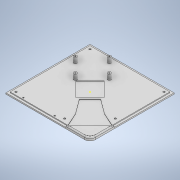
# Autodesk Inventor part: Box_Walls_2
Saved by Autodesk Inventor 2022 (Build 260153000, 153)
## iProperties
Created: 2023-02-27
Part Number: Box_Walls_2
Material: Generic
Document SubType Name: Modeling
Designer: zarek
Density: 1 g/cm^3
Appearance: Default
Author: zarek
Autodesk Inventor part; units mm, degrees
ref_plane "YZ Plane" through (0, 0, 0) normal (1, 0, 0) x (0, 1, 0)
ref_plane "XZ Plane" through (0, 0, 0) normal (0, 1, 0) x (-1, 0, 0)
sketch "Sketch1" plane through (0, 0, 0) normal (0, 1, 0) x (-1, 0, 0)
  line L0 (101.6, -101.6) -> (-101.6, -101.6)
  line L1 (-101.6, -101.6) -> (-101.6, 101.6)
  line L2 (-101.6, 101.6) -> (101.6, 101.6)
  line L3 (101.6, 101.6) -> (101.6, -101.6)
  line L4 (96.6, -96.6) -> (-96.6, -96.6)
  line L5 (-96.6, -96.6) -> (-96.6, 96.6)
  line L6 (-96.6, 96.6) -> (96.6, 96.6)
  line L7 (96.6, 96.6) -> (96.6, -96.6)
  line L8 (101.6, 101.6) -> (-40.4, 101.6)
  circle A0 centre (0, 0) radius 88.9
  circle A1 centre (0, 0) radius 109.3376
  line L9 (-40.4, 101.6) -> (-101.6, 40.4)
  line L10 (-45.4, 101.6) -> (-101.6, 45.4)
  line L11 (96.6, 96.6) -> (96.6, 101.6)
  line L12 (-45.4, 101.6) -> (-35.4, 101.6)
  line L13 (-35.4, 101.6) -> (-35.4, 96.6)
  line L14 (-35.4, 96.6) -> (-45.4, 96.6)
  line L15 (-45.4, 96.6) -> (-45.4, 101.6)
  line L16 (-45.4, 101.6) -> (-43.114, 101.6)
  line L17 (-43.114, 101.6) -> (-43.114, 96.6)
  line L18 (-43.114, 96.6) -> (-45.4, 96.6)
  line L19 (-45.4, 96.6) -> (-45.4, 101.6)
  line L20 (-96.6, 45.4) -> (-101.6, 45.4)
  line L21 (-101.6, 45.4) -> (-101.6, 43.114)
  line L22 (-101.6, 43.114) -> (-96.6, 43.114)
  line L23 (-96.6, 43.114) -> (-96.6, 45.4)
  point P0 (96.6, 51.2168)
  point P1 (101.6, 40.4)
  point P2 (101.6, -40.4)
  point P3 (96.6, -51.2168)
  point P4 (-96.6, 45.4)
  point P5 (-45.4, 96.6)
  dimension "d0" = 203.2
  dimension "d1" = 203.2
  dimension "d2" = 101.6
  dimension "d3" = 101.6
  dimension "d4" = 5
  dimension "d5" = 5
  dimension "d6" = 5
  dimension "d7" = 5
  dimension "d10" = 142
  dimension "d12" = 61.2
  dimension "d14" = 177.8
  dimension "d15" = 5
  dimension "d16" = 5
  dimension "d17" = 10
  dimension "d86" = 2.286
  dimension "d87" = 2.286
  constraints: 48 end point, 11 parallel, 10 point on line, 6 perpendicular, 5 horizontal, 2 centre point, 2 coincident, 2 point on circle
  measures "d0" distance between parallel lines of L2 L0
  measures "d1" distance between parallel lines of L1 L3
  measures "d2" distance from line of L0 point (0, 0)
  measures "d3" distance from line of L1 point (0, 0)
  measures "d4" distance between parallel lines of L4 L0
  measures "d5" distance between parallel lines of L1 L5
  measures "d6" distance between parallel lines of L2 L6
  measures "d7" distance between parallel lines of L3 L7
  measures "d10" distance of L2.end L8.end
  measures "d12" distance from line of L1 L8.end
  measures "d14" diameter of A0
  measures "d15" distance of L10.end L9.end
  measures "d16" distance of L10.start L8.end
  measures "d17" distance of L13.end L14.end
  measures "d86" distance of L17.end L18.end
  measures "d87" distance of L21.end L20.end
extrude "Extrusion1" add sketch "Sketch1" along normal blind 5 contours L0 A1 L4 L7 L3 | L0 A1 L4 | A1 L7 L3 | L0 L1 A1 L5 L4 | A1 L7 L4 | L4 A1 L5 L9 L6 L7 | A1 L7 L11 L2 L3 | L4 L5 A1 | A1 L6 L7 | L1 L9 L22 L5 A1 | L11 L6 A1 L2 | L6 L13 L2 A1 | L1 L22 A1 | A1 L22 L9 | L22 L9 L5 | L6 L17 L9 L2 L13 | L1 L20 A1 L22 | A1 L20 L9 L22 | L20 A1 L10 L5 | L5 L10 L6 L9 | A1 L17 L2 | L9 L17 A1 | L6 L9 L17 | L1 L2 L10 A1 L6 L5 | L10 A1 L20 | L10 A1 L5 | L5 A1 L6 L10 | L15 A1 L17 L9 | L6 L10 A1 L15 | L17 A1 L15 L2 | L5 L6 A1 | L6 A1 L10 | A1 L10 L15 | A0
sketch "Sketch3" plane through (0, 5, 0) normal (0, 1, 0) x (1, 0, 0)
  circle A0 centre (0, 0) radius 88.9
  line L0 (-101.6, 101.6) -> (-101.6, -101.6) projected
  line L1 (-101.6, -101.6) -> (101.6, -101.6) projected
  line L2 (-101.6, 101.6) -> (101.6, 101.6)
  line L3 (101.6, 101.6) -> (101.6, -101.6)
  line L4 (101.6, -101.6) -> (-101.6, -101.6)
  line L5 (-101.6, -101.6) -> (-101.6, 101.6)
  line L6 (-96.6, 96.6) -> (96.6, 96.6)
  line L7 (96.6, 96.6) -> (96.6, -96.6)
  line L8 (96.6, -96.6) -> (-96.6, -96.6)
  line L9 (-96.6, -96.6) -> (-96.6, 96.6)
  line L10 (-101.6, -101.6) -> (40.4, -101.6)
  circle A1 centre (0, 0) radius 109.3376
  line L11 (40.4, -101.6) -> (101.6, -40.4)
  line L12 (101.6, -101.6) -> (101.6, 101.6) projected
  line L13 (45.4038, -101.6) -> (101.6, -45.4038)
  line L14 (96.6, -45.4) -> (101.6, -45.4038)
  line L15 (45.4, -96.6) -> (45.4038, -101.6)
  line L16 (96.6, -45.4) -> (101.6, -45.4)
  line L17 (101.6, -45.4) -> (101.6, -43.114)
  line L18 (101.6, -43.114) -> (96.6, -43.114)
  line L19 (96.6, -43.114) -> (96.6, -45.4)
  line L20 (45.4038, -101.6) -> (43.1178, -101.6)
  line L21 (43.1178, -101.6) -> (43.1178, -96.6)
  line L22 (43.1178, -96.6) -> (45.4038, -96.6)
  line L23 (45.4038, -96.6) -> (45.4038, -101.6)
  point P0 (45.4038, -101.6)
  point P1 (50.4038, -96.6)
  point P2 (96.6, -50.4038)
  dimension "d28" = 177.8
  dimension "d29" = 5
  dimension "d30" = 5
  dimension "d31" = 5
  dimension "d32" = 5
  dimension "d33" = 142
  dimension "d76" = 5.0038
  dimension "d77" = 5.0038
  dimension "d88" = 2.286
  dimension "d89" = 2.286
  constraints: 42 end point, 10 point on line, 9 parallel, 4 horizontal, 4 perpendicular, 2 centre point, 2 coincident, 2 point on circle
  measures "d28" diameter of A0
  measures "d29" distance between parallel lines of L3 L7
  measures "d30" distance between parallel lines of L6 L2
  measures "d31" distance between parallel lines of L0 L9
  measures "d32" distance between parallel lines of L1 L8
  measures "d33" distance of L4.end L10.end
  measures "d76" distance of L13.end L11.end
  measures "d77" distance of L13.start L10.end
  measures "d88" distance of L17.end L16.end
  measures "d89" distance of L21.end L22.end
extrude "Extrusion3" cut sketch "Sketch3" against normal blind 2 contours L2 A1 L6 L9 L0 | A1 L9 L0 | L2 A1 L6 | A1 L9 L8 L1 L0 | L2 L3 A1 L7 L6 | A1 L8 L21 L11 L1 | L3 L11 L18 L7 A1 | A1 L21 L1 | L11 L21 A1 | L3 L18 A1 | A1 L18 L11
sketch "Sketch4" plane through (0, 5, 0) normal (0, 1, 0) x (1, 0, 0)
  line L0 (101.6, 101.6) -> (-101.6, 101.6)
  line L1 (-101.6, 101.6) -> (-101.6, -101.6)
  line L2 (-101.6, -101.6) -> (101.6, -101.6)
  line L3 (101.6, -101.6) -> (101.6, 101.6)
  circle A0 centre (0, 0) radius 2.5
  line L4 (11.3314, 2.139) -> (-2.139, -11.3314)
  line L5 (0, 0) -> (-5.6569, 5.6569)
  line L6 (-5.6569, -14.8492) -> (-26.163, 5.6569)
  line L7 (-5.6569, 26.163) -> (14.8492, 5.6569)
  circle A1 centre (-5.6569, 5.6569) radius 14
  line L8 (-26.163, 5.6569) -> (-5.6569, 26.163)
  line L9 (14.8492, 5.6569) -> (-5.6569, -14.8492)
  line L10 (-40.3051, 5.6569) -> (-5.6569, 40.3051)
  line L11 (-5.6569, 40.3051) -> (28.9914, 5.6569)
  line L12 (28.9914, 5.6569) -> (-5.6569, -28.9914)
  line L13 (-5.6569, -28.9914) -> (-40.3051, 5.6569)
  line L14 (-22.6451, 9.1747) -> (-9.1747, 22.6451)
  line L15 (-9.1747, 22.6451) -> (-12.7668, 26.2372)
  line L16 (-12.7668, 26.2372) -> (-26.2372, 12.7668)
  line L17 (-26.2372, 12.7668) -> (-22.6451, 9.1747)
  point P0 (9.525, 22.5)
  point P1 (-9.525, -6.5)
  dimension "d37" = 203.2
  dimension "d38" = 203.2
  dimension "d39" = 8
  dimension "d40" = 28
  dimension "d41" = 29
  dimension "d42" = 29
  dimension "d43" = 14.5
  dimension "d44" = 10
  dimension "d45" = 10
  dimension "d46" = 10
  dimension "d47" = 10
  dimension "d48" = 5.08
  dimension "d49" = 9.525
  dimension "d50" = 9.525
  dimension "d55" = 101.6
  dimension "d56" = 101.6
  constraints: 36 end point, 8 parallel, 4 perpendicular, 2 centre point, 2 coincident, 2 point on line, 1 horizontal
  measures "d37" distance between parallel lines of L2 L0
  measures "d38" distance between parallel lines of L1 L3
  measures "d39" distance of L5.start L5.end
  measures "d40" diameter of A1
  measures "d41" distance between parallel lines of L9 L8
  measures "d42" distance between parallel lines of L7 L6
  measures "d43" distance from line of A1.centre L8
  measures "d44" distance between parallel lines of L11 L7
  measures "d45" distance between parallel lines of L8 L10
  measures "d46" distance between parallel lines of L13 L6
  measures "d47" distance between parallel lines of L12 L9
  measures "d48" distance between parallel lines of L14 L16
  measures "d49" distance from line of A1.centre L15
  measures "d50" distance from line of L5.end L17
  measures "d55" distance from line of point (0, 0) L1
  measures "d56" distance from line of L0 point (0, 0)
extrude "Extrusion4" cut sketch "Sketch4" against normal blind 1 contours A0 | L4 L9 L6 L8 L7 | L8 L17 L16 L15 | A1 | L10 L11 L12 L13
sketch "Sketch6" plane through (0, 5, 0) normal (0, 1, 0) x (1, 0, 0)
  line L0 (45.4038, -101.6) -> (0, 0)
  line L1 (50.4038, -96.6) -> (45.4038, -101.6) projected
  line L2 (96.6, -43.114) -> (96.6, 96.6) projected
  line L3 (101.6, -101.6) -> (101.6, 101.6) projected
  circle A0 centre (0, 0) radius 34.925
  circle A1 centre (0, 0) radius 33.425
  line L4 (-101.6, 101.6) -> (-101.6, -101.6) projected
  line L5 (-101.6, -101.6) -> (40.4, -101.6)
  line L6 (-101.6, -101.6) -> (101.6, -101.6) projected
  line L7 (101.6, 101.6) -> (101.6, -43.114) projected
  line L8 (101.6, -45.4038) -> (0, 0)
  line L9 (-96.6, -96.6) -> (43.1178, -96.6) projected
  line L10 (96.6, -43.114) -> (96.6, 96.6) projected
  line L11 (43.1178, -101.6) -> (-101.6, -101.6) projected
  line L12 (101.6, -45.4038) -> (96.6, -50.4038) projected
  line L13 (45.4038, -101.6) -> (101.6, -45.4038)
  line L14 (43.1178, -101.6) -> (101.6, -101.6) projected
  line L15 (0, 0) -> (101.6, -50.4076)
  line L16 (50.4076, -101.6) -> (0, 0)
  line L17 (43.1694, -96.6) -> (47.9269, -96.6)
  line L18 (96.6, -43.1694) -> (96.6, -47.9269)
  line L19 (40.4, -101.6) -> (101.6, -40.4)
  point P0 (13.6374, -30.5164)
  point P1 (30.5164, -13.6374)
  point P2 (14.2494, -31.8859)
  point P3 (31.2861, -15.5222)
  point P4 (29.9423, -14.8555)
  point P5 (31.8859, -14.2494)
  point P6 (98.2555, -48.7483)
  point P7 (96.6, -47.9269)
  point P8 (47.9269, -96.6)
  point P9 (15.5222, -31.2861)
  point P10 (96.6, -45.4)
  point P11 (45.4, -96.6)
  point P12 (14.8555, -29.9423)
  point P13 (96.6, -45.4)
  point P14 (45.4, -96.6)
  point P15 (45.4, -96.6)
  point P16 (47.089, -94.911)
  point P17 (94.911, -47.089)
  point P18 (96.6, -45.4)
  point P19 (43.8583, -98.1417)
  point P20 (98.1417, -43.8583)
  point P21 (45.4, -96.6)
  point P22 (96.6, -45.4)
  dimension "d71" = 69.85
  dimension "d72" = 66.85
  dimension "d75" = 142
  dimension "d78" = 5.0038
  dimension "d82" = 5.0038
  constraints: 18 end point, 11 point on line, 2 centre point, 2 coincident, 1 collinear, 1 perpendicular
  measures "d71" diameter of A0
  measures "d72" diameter of A1
  measures "d75" distance of L4.end L5.end
  measures "d78" distance of L0.start L5.end
  measures "d82" distance of L8.start L19.end
extrude "Extrusion6" cut sketch "Sketch6" against normal blind 1 contours L0 A0 L16 L19 L17 | L0 A1 L16 A0 | L16 A1 L15 A0 | L15 A0 L8 L18 L19 | A0 L15 A1 L8
sketch "Sketch8" plane through (0, 5, 0) normal (0, 1, 0) x (1, 0, 0)
  line L0 (101.6, -101.6) -> (101.6, 101.6) projected
  line L1 (-96.6, -96.6) -> (43.1178, -96.6) projected
  line L2 (101.6, -101.6) -> (43.1178, -101.6)
  line L3 (43.1178, -101.6) -> (43.1178, -96.6)
  line L4 (43.1178, -96.6) -> (101.6, -96.6)
  line L5 (101.6, -96.6) -> (101.6, -101.6)
  line L6 (96.6, -43.114) -> (96.6, 96.6) projected
  line L7 (101.6, -101.6) -> (96.6, -101.6)
  line L8 (96.6, -101.6) -> (96.6, -43.114)
  line L9 (96.6, -43.114) -> (101.6, -43.114)
  line L10 (101.6, -43.114) -> (101.6, -101.6)
  line L11 (96.6, -45.4) -> (94.911, -47.089) projected
  line L12 (15.5222, -31.2861) -> (47.089, -94.911) projected
  line L13 (43.1178, -101.6) -> (101.6, -101.6) projected
  line L14 (43.1178, -101.6) -> (-101.6, -101.6) projected
  line L15 (-101.6, -101.6) -> (40.4, -101.6)
  line L16 (101.602, -101.6048) -> (-101.598, -101.6048)
  line L17 (-101.598, -101.6048) -> (-101.598, 101.5952)
  line L18 (-101.598, 101.5952) -> (101.602, 101.5952)
  line L19 (101.602, 101.5952) -> (101.602, -101.6048)
  line L20 (96.602, -96.6048) -> (-96.598, -96.6048)
  line L21 (-96.598, -96.6048) -> (-96.598, 96.5952)
  line L22 (-96.598, 96.5952) -> (96.602, 96.5952)
  line L23 (96.602, 96.5952) -> (96.602, -96.6048)
  line L24 (101.602, 101.5952) -> (-40.398, 101.5952)
  circle A0 centre (0.002, -0.0048) radius 88.9
  circle A1 centre (0.002, -0.0048) radius 109.3376
  line L25 (-40.398, 101.5952) -> (-101.598, 40.3952)
  line L26 (-45.398, 101.5952) -> (-101.598, 45.3952)
  line L27 (96.602, 96.5952) -> (96.602, 101.5952)
  line L28 (-45.398, 101.5952) -> (-35.398, 101.5952)
  line L29 (-35.398, 101.5952) -> (-35.398, 96.5952)
  line L30 (-35.398, 96.5952) -> (-45.398, 96.5952)
  line L31 (-45.398, 96.5952) -> (-45.398, 101.5952)
  line L32 (43.1178, -96.6) -> (43.1178, -101.6) projected
  line L33 (43.1178, -100.4824) -> (43.1178, -101.6)
  line L34 (51.2188, -96.6048) -> (52.3364, -96.6048)
  line L35 (100.4824, -43.114) -> (101.6, -43.114)
  line L36 (96.602, -51.2216) -> (96.602, -52.3392)
  line L37 (43.1178, -101.6) -> (46.9278, -101.6048)
  line L38 (101.6, -43.114) -> (101.602, -46.924)
  line L39 (101.602, -46.924) -> (96.602, -52.4916)
  line L40 (96.602, -51.2216) -> (96.602, -54.3174)
  line L41 (46.9278, -101.6048) -> (52.4888, -96.6048)
  line L42 (51.2188, -96.6048) -> (52.4888, -96.6048)
  point P0 (0, 0)
  point P1 (-96.598, -96.6)
  point P2 (43.1178, -96.6048)
  point P3 (101.6, -46.9262)
  point P4 (46.9332, -101.6)
  dimension "d93" = 142
  dimension "d94" = 203.2
  dimension "d95" = 203.2
  dimension "d96" = 101.6
  dimension "d97" = 101.6
  dimension "d98" = 5
  dimension "d99" = 5
  dimension "d100" = 5
  dimension "d101" = 5
  dimension "d102" = 142
  dimension "d103" = 61.2
  dimension "d104" = 177.8
  dimension "d105" = 5
  dimension "d106" = 5
  dimension "d107" = 10
  dimension "d116" = 3.81
  dimension "d117" = 3.81
  dimension "d118" = 1.27
  dimension "d119" = 1.27
  constraints: 70 end point, 17 point on line, 13 parallel, 6 perpendicular, 6 point on circle, 5 horizontal, 2 centre point, 2 coincident, 2 collinear, 1 vertical
  measures "d93" distance of L14.end L15.end
  measures "d94" distance between parallel lines of L18 L16
  measures "d95" distance between parallel lines of L17 L19
  measures "d96" distance from line of L16 point (0.002, -0.005)
  measures "d97" distance from line of L17 point (0.002, -0.005)
  measures "d98" distance between parallel lines of L20 L16
  measures "d99" distance between parallel lines of L17 L21
  measures "d100" distance between parallel lines of L18 L22
  measures "d101" distance between parallel lines of L19 L23
  measures "d102" distance of L24.start L24.end
  measures "d103" distance from line of L17 L24.end
  measures "d104" diameter of A0
  measures "d105" distance of L26.end L25.end
  measures "d106" distance of L31.end L24.end
  measures "d107" distance of L30.start L31.start
  measures "d116" distance of L2.end L37.end
  measures "d117" distance of L9.end L38.end
  measures "d118" distance of L39.end L36.start
  measures "d119" distance of L41.end L34.start
extrude "Extrusion7" add sketch "Sketch8" along normal blind 3 contours L2 L8 L4 L0 | L4 L8 L39 L0 | L2 L41 L20 L8
fillet "Fillet3" radius 12.7 2 edges at (101.6, 4, 101.6) (96.602, 6.5, 96.6048)
fillet "Fillet4" radius 3.175 6 edges at (97.8803, 8, 97.8803) (101.6, 8, 67.9131) (67.9166, 8, 101.6) (92.8822, 8, 92.8851) (96.602, 8, 68.1982) (68.1954, 8, 96.6048)
sketch "Sketch9" plane through (0, 4, 0) normal (0, 1, 0) x (1, 0, 0)
  point P0 (0, 0)
sketch "Sketch10" plane through (0, 5, 0) normal (0, 1, 0) x (1, 0, 0)
  point P0 (0, 0)
ref_plane "Work Plane1" through (24.6957, 5, 24.6957) normal (0.7071068, 0, 0.7071068) x (0.7071068, 0, -0.7071068)
sketch "Sketch15" plane through (0, 5, 0) normal (0, 1, 0) x (1, 0, 0)
  line L0 (43.1694, -96.6) -> (13.6374, -30.5164) projected
  line L1 (28.4034, -63.5582) -> (-0.6569, -23.9914)
  line L2 (28.9914, 5.6569) -> (-5.6569, -28.9914) projected
  line L3 (30.5164, -13.6374) -> (96.6, -43.1694) projected
  line L4 (-5.6569, 40.3051) -> (28.9914, 5.6569) projected
  line L5 (63.5582, -28.4034) -> (23.9914, 0.6569)
  line L6 (2.3374, -28.0682) -> (28.0682, -2.3374)
  arc A0 (13.6374, -30.5164) -> (30.5164, -13.6374) centre (0, 0) ccw projected
  line L7 (28.4034, -63.5582) -> (13.6374, -30.5164)
  line L8 (63.5582, -28.4034) -> (30.5164, -13.6374)
  arc A1 (13.6374, -30.5164) -> (30.5164, -13.6374) centre (0, 0) ccw
  line L9 (28.6195, -64.3953) -> (1.6303, -28.7753)
  line L10 (1.6303, -28.7753) -> (2.3374, -28.0682)
  dimension "d138" = 5
  dimension "d139" = 5
  dimension "d140" = 5
  dimension "d168" = 1
  constraints: 14 end point, 4 point on line, 3 point on circle, 2 midpoint, 1 centre point, 1 collinear, 1 concentric, 1 parallel
  measures "d138" horizontal distance of L2.end L1.end
  measures "d139" horizontal distance of L2.start L5.end
  measures "d140" distance between parallel lines of L6 L2
  measures "d168" distance of L6.start L9.end
extrude "Extrusion11" cut sketch "Sketch15" against normal blind 1 contours L1 L6 L5 L3 A0 L0
sketch "Sketch16" plane through (0, 4, 0) normal (0, 1, 0) x (1, 0, 0)
  line L0 (2.3374, -28.0682) -> (28.0682, -2.3374) projected
  line L1 (9.4085, -20.9971) -> (12.944, -24.5327)
  line L2 (12.944, -24.5327) -> (24.5327, -12.944)
  line L3 (24.5327, -12.944) -> (20.9971, -9.4085)
  line L4 (12.944, -24.5327) -> (24.5327, -12.944)
  line L5 (24.5327, -12.944) -> (28.5592, -16.9706)
  line L6 (28.5592, -16.9706) -> (16.9706, -28.5592)
  line L7 (16.9706, -28.5592) -> (12.944, -24.5327)
  line L8 (12.944, -24.5327) -> (5.3317, -32.145)
  line L9 (28.4034, -63.5582) -> (2.3374, -28.0682) projected
  line L10 (24.5327, -12.944) -> (32.145, -5.3317)
  line L11 (28.0682, -2.3374) -> (63.5582, -28.4034) projected
  point P0 (0, 0)
  dimension "d144" = 10
  dimension "d145" = 10
  dimension "d146" = 5
  dimension "d152" = 0
  dimension "d153" = 0
  constraints: 18 end point, 6 perpendicular, 6 point on line
  measures "d144" distance of L0.start L1.start
  measures "d145" distance of L0.end L3.end
  measures "d146" distance between parallel lines of L0 L2
  measures "d152" distance between parallel lines of L7 L1
  measures "d153" distance between parallel lines of L5 L3
extrude "Extrusion12" cut sketch "Sketch16" along normal up to surface (1 mm away)
sketch "Sketch20" plane through (0, 5, 0) normal (0, 1, 0) x (1, 0, 0)
  line L0 (47.089, -94.911) -> (45.4, -96.6) projected
  line L1 (47.089, -94.911) -> (94.9376, -47.0624)
  line L2 (94.1649, -47.8351) -> (33.507, -17.7404)
  line L3 (94.911, -47.089) -> (31.2861, -15.5222) projected
  line L4 (15.5222, -31.2861) -> (47.089, -94.911) projected
  line L5 (17.5265, -33.0758) -> (47.8351, -94.1649)
  arc A0 (15.5222, -31.2861) -> (31.2861, -15.5222) centre (0, 0) ccw projected
  line L6 (33.507, -17.7404) -> (31.7193, -16.8534)
  line L7 (17.5265, -33.0758) -> (16.7531, -31.5169)
  arc A1 (16.7531, -31.5169) -> (31.7193, -16.8534) centre (3.7904, -3.3173) ccw
  dimension "d169" = 1
  dimension "d172" = 1
  constraints: 10 end point, 2 point on circle, 2 point on line, 1 centre point, 1 collinear, 1 parallel
  measures "d169" distance between parallel lines of L2 L3
  measures "d172" distance between parallel lines of L5 L4
extrude "Extrusion13" cut sketch "Sketch20" against normal blind 1 contours L4 A0 L3 L1 L2 L6 A1 L7 L5
sketch "Sketch21" plane through (0, 5, 0) normal (0, 1, 0) x (1, 0, 0)
  line L0 (47.8351, -94.1649) -> (45.4, -96.6) projected
  line L1 (47.8351, -94.1649) -> (94.1583, -47.8417)
  arc A0 (16.7531, -31.5169) -> (31.7193, -16.8534) centre (3.7904, -3.3173) ccw projected
  line L2 (31.7193, -16.8534) -> (16.7531, -31.5169)
  line L3 (16.7531, -31.5169) -> (47.8351, -94.1649)
  line L4 (96.6, -45.4) -> (94.1649, -47.8351) projected
  line L5 (94.1649, -47.8351) -> (94.1583, -47.8417)
  arc A1 (16.7531, -31.5169) -> (31.7193, -16.8534) centre (3.7904, -3.3173) ccw projected
  line L6 (94.1649, -47.8351) -> (31.7193, -16.8534)
  point P0 (0, 0)
  constraints: 10 end point, 2 collinear
extrude "Extrusion14" cut sketch "Sketch21" against normal blind 1 contours L3 A0 L6 L5 L1
sketch "Sketch22" plane through (0, 5, 0) normal (0, 1, 0) x (1, 0, 0)
  point P0 (0, 0)
sketch "Sketch23" plane through (0, 5, 0) normal (0, 1, 0) x (1, 0, 0)
  circle A0 centre (0.3398, -3.529) radius 1.3882
  circle A1 centre (58.5491, -3.529) radius 1.3899
  circle A2 centre (58.5491, -52.5159) radius 1.3668
  circle A3 centre (0.3398, -52.5159) radius 1.3668
  line L0 (82, -53) -> (82, -3)
  line L1 (-3, -3) -> (-3, -53)
  line L2 (0.0454, -57.893) -> (79, -56)
  line L3 (81.1565, 1.9458) -> (0, 0)
  line L4 (0, 0) -> (-26.9408, 26.9408)
  line L5 (0, 0) -> (0, 43.6117)
  line L6 (-26.9408, 26.9408) -> (-3.6062, 50.2753)
  line L7 (-38.2545, 84.9235) -> (-79.2667, 43.9113)
  line L8 (-79.2667, 43.9113) -> (-44.6184, 9.2631)
  line L9 (-44.6184, 9.2631) -> (-26.9408, 26.9408)
  line L10 (-26.9408, 26.9408) -> (-61.589, 61.589)
  line L11 (-38.2545, 84.9235) -> (-3.6062, 50.2753)
  circle A4 centre (-38.2545, 84.9235) radius 4
  circle A5 centre (-3.6062, 50.2753) radius 4
  circle A6 centre (-79.2667, 43.9113) radius 4
  circle A7 centre (-44.6184, 9.2631) radius 4
  point P0 (39.5, -28)
  dimension "d178" = 48.9869
  dimension "d179" = 48.9869
  dimension "d180" = 58.2093
  dimension "d181" = 85
  dimension "d182" = 57.8775
  dimension "d183" = 38.1
  dimension "d184" = 45
  dimension "d187" = 33
  dimension "d188" = 25
  dimension "d189" = 49
  dimension "d190" = 8
  dimension "d191" = 8
  dimension "d192" = 8
  dimension "d193" = 8
  constraints: 24 end point, 8 centre point, 5 coincident, 4 perpendicular, 2 parallel, 1 point on line, 1 vertical
  measures "d178" distance of A3.centre A0.centre
  measures "d179" distance of A2.centre A1.centre
  measures "d180" distance of A0.centre A1.centre
  measures "d181" distance between parallel lines of L0 L1
  measures "d182" distance between parallel lines of L2 L3
  measures "d183" distance of L3.end L4.end
  measures "d184" angle of L4 L5
  measures "d187" distance between parallel lines of L10 L11
  measures "d188" distance between parallel lines of L8 L10
  measures "d189" distance between parallel lines of L6 L7
  measures "d190" diameter of A4
  measures "d191" diameter of A5
  measures "d192" diameter of A6
  measures "d193" diameter of A7
extrude "Extrusion15" add sketch "Sketch23" along normal blind 12.7 contours A5 L11 L6 | L6 L11 A5 | A7 L8 L9 | L9 L8 A7 | A4 L11 L7 | L7 L11 A4 | A6 L8 L7 | L7 L8 A6
sketch "Sketch24" plane through (-44.6184, 17.7, -9.2631) normal (0, 1, 0) x (1, 0, 0)
  circle A0 centre (0, 0) radius 4
  circle A1 centre (41.0122, 41.0122) radius 4 projected
  circle A2 centre (41.0122, 41.0122) radius 4
  circle A3 centre (-34.8079, 34.6819) radius 3.9695
  circle A4 centre (6.332, 75.5141) radius 4.1464
  point P0 (44.6184, -9.2631)
  constraints: 4 centre point, 1 coincident
hole "Hole2" at (-79.4263, 17.7, -43.945) at (-44.6184, 17.7, -9.2631) at (-38.2865, 17.7, -84.7772) at (-3.6062, 17.7, -50.2753) direction (0, -1, 0) diameter 2.85 depth 12.7 tip angle 118 countersink diameter 3.175 countersink angle 82 thread size "M3.5x0.6" class "6H" standard "ANSI Metric M Profile"
sketch "Sketch25" plane through (0, 5, 0) normal (0, 1, 0) x (1, 0, 0)
  line L0 (-96.6, 96.6) -> (-96.6, -96.6) projected
  line L1 (96.6, 96.6) -> (-96.6, 96.6) projected
  line L2 (-96.6, 96.6) -> (96.6, 96.6)
  line L3 (96.6, -45.4) -> (45.4, -96.6) projected
  line L4 (96.6, 96.6) -> (96.6, -45.4)
  line L5 (96.6, -45.4) -> (45.4, -96.6)
  line L6 (45.4, -96.6) -> (-96.6, -96.6)
  line L7 (-96.6, -96.6) -> (-96.6, 96.6)
  line L8 (-96.6, 96.6) -> (-89.5289, 89.5289)
  circle A0 centre (-89.5289, 89.5289) radius 5
  circle A1 centre (-89.5289, 89.5289) radius 1.5
  line L9 (-89.5289, 84.5289) -> (-96.6, 84.5289)
  line L10 (-89.5289, 89.5289) -> (-89.5289, 84.5289)
  line L11 (-89.5289, 89.5289) -> (-84.5289, 89.5289)
  line L12 (-84.5289, 96.6) -> (-84.5289, 89.5289)
  line L13 (-96.6, -96.6) -> (-89.5289, -89.5289)
  line L14 (-96.6, -96.6) -> (-86.6, -96.6) construction
  circle A2 centre (-89.5289, -89.5289) radius 5
  circle A3 centre (-89.5289, -89.5289) radius 1.75
  line L15 (-89.5289, -89.5289) -> (-84.5289, -89.5289)
  line L16 (-84.5289, -96.6) -> (-84.5289, -89.5289)
  line L17 (-89.5289, -89.5289) -> (-89.5289, -84.5289)
  line L18 (-96.6, -84.5289) -> (-89.5289, -84.5289)
  line L19 (96.6, 96.6) -> (89.5289, 89.5289)
  circle A4 centre (89.5289, 89.5289) radius 5
  circle A5 centre (89.5289, 89.5289) radius 1.75
  line L20 (89.5289, 89.5289) -> (84.5289, 89.5289)
  line L21 (84.5289, 96.6) -> (84.5289, 89.5289)
  line L22 (89.5289, 89.5289) -> (89.5289, 84.5289)
  line L23 (96.6, 84.5289) -> (89.5289, 84.5289)
  line L24 (96.6, -43.114) -> (96.6, 96.6) projected
  line L25 (-96.6, -96.6) -> (43.1178, -96.6) projected
  line L26 (28.9914, 5.6569) -> (-5.6569, -28.9914) projected
  line L27 (25.4, -25.4) -> (101.6, -25.4)
  line L28 (101.6, -88.9) -> (101.6, 101.6) projected
  line L29 (25.4, -25.4) -> (25.4, -101.6)
  line L30 (43.1178, -101.6) -> (-101.6, -101.6) projected
  line L31 (96.6, -25.4) -> (86.6, -25.4)
  circle A6 centre (86.6, -25.4) radius 5
  circle A7 centre (86.6, -25.4) radius 1.75
  line L32 (25.4, -96.6) -> (25.4, -86.6)
  circle A8 centre (25.4, -86.6) radius 5
  circle A9 centre (25.4, -86.6) radius 1.75
  point P0 (0, 0)
  dimension "d203" = 10
  dimension "d205" = 3
  dimension "d206" = 10
  dimension "d207" = 45
  dimension "d208" = 10
  dimension "d209" = 3.5
  dimension "d210" = 10
  dimension "d211" = 10
  dimension "d212" = 3.5
  dimension "d223" = 76.2
  dimension "d224" = 76.2
  dimension "d225" = 10
  dimension "d226" = 10
  dimension "d227" = 3.5
  dimension "d228" = 10
  dimension "d229" = 10
  dimension "d230" = 3.5
  constraints: 50 end point, 14 point on line, 10 centre point, 9 coincident, 9 perpendicular, 6 point on circle, 5 horizontal, 3 parallel, 2 tangent, 1 collinear, 1 equal length, 1 vertical
  measures "d203" distance of L0.start L8.end
  measures "d205" diameter of A1
  measures "d206" distance of L6.end L13.end
  measures "d207" angle of L14 L13
  measures "d208" diameter of A2
  measures "d209" diameter of A3
  measures "d210" distance of L1.start L19.end
  measures "d211" diameter of A4
  measures "d212" diameter of A5
  measures "d223" distance between parallel lines of L28 L29
  measures "d224" distance between parallel lines of L30 L27
  measures "d225" distance of L31.start L31.end
  measures "d226" diameter of A6
  measures "d227" diameter of A7
  measures "d228" distance of L32.start L32.end
  measures "d229" diameter of A8
  measures "d230" diameter of A9
hole "Hole3" at (-89.5289, 5, 89.5289) at (-89.5289, 5, -89.5289) at (89.5289, 5, -89.5289) at (25.4, 5, 86.6) at (86.6, 5, 25.4) direction (0, -1, 0) diameter 2.85 depth 12.7 tip angle 118 countersink diameter 4.445 countersink angle 82 thread size "M3.5x0.6" class "6H" standard "ANSI Metric M Profile"
sketch "Sketch26" plane through (0, 5, 0) normal (0, 1, 0) x (1, 0, 0)
  line L0 (-96.6, -92.6793) -> (-96.6, -59.6793)
  line L1 (-68.6, -92.6793) -> (-96.6, -92.6793)
  line L2 (-96.6, -96.6) -> (43.1178, -96.6) projected
  line L3 (-68.6, -92.6793) -> (-68.6, -96.6)
  line L4 (-68.6, -92.6793) -> (7.4, -92.6793)
  circle A0 centre (-68.6, -92.6793) radius 1.5
  circle A1 centre (7.4, -92.6793) radius 1.5
  line L5 (-101.6, -101.6) -> (-101.6, 101.6) projected
  point P0 (0, 0)
  dimension "d232" = 3.9207
  dimension "d234" = 76
  dimension "d235" = 3
  dimension "d236" = 3
  dimension "d244" = 33
  constraints: 8 end point, 2 centre point, 2 coincident, 2 horizontal, 1 perpendicular, 1 point on line
  measures "d232" distance between parallel lines of L2 L1
  measures "d234" distance of L1.start L4.end
  measures "d235" diameter of A0
  measures "d236" diameter of A1
  measures "d244" distance from line of L5 L1.start
hole "Hole4" at (-68.6, 5, 92.6793) at (7.4, 5, 92.6793) direction (0, -1, 0) diameter 2.85 depth 2.54 tip angle 118 countersink diameter 3.175 countersink angle 82 thread size "M3.5x0.6" class "6H" standard "ANSI Metric M Profile"
sketch "Sketch27" plane through (0, 5, 0) normal (0, 1, 0) x (1, 0, 0)
  point P0 (0, 0)
equation "\"d1\" = d0"
equation "\"d2\" = 0.5 * d0"
equation "\"d3\" = 0.5 * d0"
equation "\"d95\" = d94"
equation "\"d96\" = 0.5 * d94"
equation "\"d97\" = 0.5 * d94"
body "Solid1"
